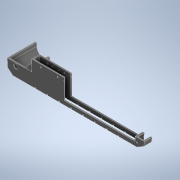
# Autodesk Inventor part: dolni-cast
Saved by Autodesk Inventor 2022 (Build 260153000, 153)
## iProperties
Created: 2022-11-08
Part Number: dolni-cast
Material: Generic
Document SubType Name: Modeling
Designer: matys
Density: 1 g/cm^3
Appearance: Gray
Author: matys
Autodesk Inventor part; units mm, degrees
ref_plane "YZ Plane" through (0, 0, 0) normal (1, 0, 0) x (0, 1, 0)
ref_plane "XZ Plane" through (0, 0, 0) normal (0, 1, 0) x (-1, 0, 0)
ref_plane "XY Plane" through (0, 0, 0) normal (0, 0, 1) x (1, 0, 0)
sketch "Sketch1" plane through (0, 0, 0) normal (0, 1, 0) x (-1, 0, 0)
  line L0 (0, 0) -> (0, -100)
  line L1 (0, 0) -> (-247.347, 0)
  line L2 (-247.347, 0) -> (-247.347, -100)
  line L3 (-247.347, -100) -> (0, -100)
  dimension "d0" = 100
  dimension "d1" = 247.347
  dimension "d2" = 100
  constraints: 8 end point, 1 horizontal, 1 perpendicular, 1 vertical
  measures "d0" distance of L0.start L0.end
  measures "d1" distance of L0.start L1.end
  measures "d2" distance of L1.end L2.end
extrude "Extrusion1" add sketch "Sketch1" along normal blind 38.0143
sketch "Sketch2" plane through (0, 0, 0) normal (0, 0, 1) x (1, 0, 0)
  line L0 (247.347, 0) -> (0, 0)
  line L1 (0, 0) -> (0, 3.5)
  line L2 (0, 0) -> (0, 38.0143)
  line L3 (247.347, 0) -> (247.347, 38.0143)
  line L4 (0, 3.5) -> (2, 3.5)
  line L5 (0, 0) -> (0, 3.5)
  line L6 (0, 3.5) -> (2, 3.5)
  line L7 (247.347, 38.0143) -> (0, 38.0143)
  arc A0 (3.965119, 16.034845) -> (16.530008, 3.5) centre (16.5, 16.034845) ccw
  line L8 (16.5, 16.034845) -> (3.965119, 16.034845)
  line L9 (2, 16.034845) -> (2, 8.034845)
  line L10 (6.849962, 8.034845) -> (14.857533, 8.034845)
  line L11 (14.857533, 8.034845) -> (6.849962, 8.034845)
  line L12 (2, 8.034845) -> (11.575556, 0)
  line L13 (2, 16.034845) -> (0, 38.0143)
  line L14 (2, 3.5) -> (7.404418, 3.5)
  line L15 (16.469992, 3.5) -> (16.530008, 3.5)
  line L16 (0, 3.5) -> (7.404418, 3.5)
  line L17 (2, 16.034845) -> (3, 16.034845)
  line L18 (1.663936, 35.652509) -> (1.493828, 38.15023)
  line L19 (3.094685, 35.782699) -> (1.663936, 35.652509)
  line L20 (0, 38.0143) -> (1.493828, 38.15023)
  line L21 (3.094685, 35.782699) -> (3.965119, 16.034845)
  line L22 (247.347, 0) -> (230.9326, 0)
  line L23 (230.9326, 0) -> (230.9326, 3.5)
  line L24 (230.9326, 3.5) -> (242.883751, 10.4)
  line L25 (231.248952, 0.023376) -> (243.200103, 6.923376)
  line L26 (243.200103, 6.923376) -> (247.347, 25.567765)
  line L27 (240.6078, 9.085979) -> (243.787005, 23.379642)
  line L28 (244.329151, 25.817122) -> (247.347, 25.817122)
  line L29 (16.469992, 3.5) -> (230.9326, 3.5)
  line L30 (237.270641, 3.5) -> (247.347, 3.5)
  line L31 (247.347, 25.567765) -> (247.347, 25.817122)
  line L32 (244.329151, 25.817122) -> (245.829151, 25.817122)
  line L33 (245.829151, 25.817122) -> (245.273551, 23.379642)
  line L34 (245.273551, 23.379642) -> (243.787005, 23.379642)
  line L35 (247.347, 25.567765) -> (247.347, 0)
  line L36 (231.208463, 0) -> (247.347, 0)
  line L37 (247.347, 25.817122) -> (247.347, 38.0143)
  line L38 (247.347, 38.0143) -> (1.503086, 38.0143)
  line L39 (0, 38.0143) -> (0, 0)
  line L40 (0, 0) -> (11.575556, 0)
  line L41 (11.575556, 0) -> (231.208463, 0)
  line L42 (231.248952, 0.023376) -> (231.208463, 0)
  point P0 (16.530008, 3.5)
  dimension "d5" = 3.5
  dimension "d9" = 2
  dimension "d12" = 8
  dimension "d13" = 12.5
  dimension "d14" = 40
  dimension "d17" = 1
  dimension "d20" = 16.4144
  dimension "d21" = 13.8
  dimension "d23" = 13.8
  dimension "d24" = 19.1
  dimension "d26" = 17.14
  dimension "d27" = 1.5
  dimension "d28" = 2.5
  constraints: 78 end point, 15 point on line, 10 collinear, 6 horizontal, 5 perpendicular, 4 point on circle, 2 parallel, 1 centre point
  measures "d5" distance of L0.end L1.end
  measures "d9" distance of L1.end L4.end
  measures "d12" distance of L9.start L9.end
  measures "d13" distance of L9.end L12.end
  measures "d14" angle of L10 L12
  measures "d17" distance of L9.start L17.end
  measures "d20" distance of L0.start L22.end
  measures "d21" distance of L23.end L24.end
  measures "d23" distance of L25.start L25.end
  measures "d24" distance of L25.end L26.end
  measures "d26" distance of L27.start L28.start
  measures "d27" distance of L28.start L32.end
  measures "d28" distance of L32.end L33.end
extrude "Extrusion2" cut sketch "Sketch2" against normal through all contours L0 L42 L25 L30 L3 | L30 L25 L26 L3 | L0 L1 L4 L14 L12 | L29 A0 L21 L19 L18 L7 L3 L28 L33 L34 L27 L24 | L14 L4 L2 L13 L9 L12
sketch "Sketch3" plane through (16.469992, 3.5, 0) normal (0, 1, 0) x (1, 0, 0)
  line L0 (226.73011, 0) -> (230.877008, 0)
  line L1 (230.877008, 0) -> (230.877008, 2)
  line L2 (230.877008, 0) -> (230.877008, 100)
  line L3 (230.877008, 2) -> (-16.469992, 2)
  line L4 (-16.469992, 100) -> (-16.469992, 0)
  line L5 (-16.469992, 0) -> (-16.469992, 2)
  line L6 (-16.469992, 0) -> (-14.966906, 0)
  line L7 (-16.469992, 0) -> (230.877008, 0)
  line L8 (230.877008, 0) -> (230.877008, 100)
  line L9 (230.877008, 100) -> (-16.469992, 100)
  line L10 (-16.469992, 100) -> (-16.469992, 98)
  line L11 (-16.469992, 98) -> (230.877008, 98)
  line L12 (230.877008, 100) -> (230.877008, 98)
  point P0 (226.73011, 0)
  dimension "d31" = 2
  dimension "d32" = 2
  constraints: 18 end point, 5 perpendicular, 5 point on line, 1 collinear
  measures "d31" distance of L0.end L1.end
  measures "d32" distance of L9.end L10.end
extrude "Extrusion3" add sketch "Sketch3" along normal blind 34.5143 contours L7 L6 L4 L3 L1 L0 | L11 L4 L9 L2
sketch "Sketch4" plane through (0, 3.5, -98) normal (0, 0, 1) x (1, 0, 0)
  line L0 (11.575556, -3.5) -> (7.404418, 0)
  line L1 (7.404418, 0) -> (2, 4.534845)
  line L2 (7.404418, 0) -> (2, 4.534845)
  line L3 (2, 4.534845) -> (2, 12.534845)
  line L4 (2, 4.534845) -> (2, 12.534845)
  line L5 (2, 12.534845) -> (0, 34.5143)
  line L6 (2, 12.534845) -> (0, 34.5143)
  line L7 (0, 0) -> (0, 34.5143)
  line L8 (0, 34.5143) -> (0, 0)
  line L9 (0, 0) -> (7.404418, 0)
  point P0 (0, -3.5)
  constraints: 10 end point, 4 collinear, 1 perpendicular
extrude "Extrusion4" cut sketch "Sketch4" along normal through all both and the other way through all
sketch "Sketch5" plane through (237.270641, 3.5, -98) normal (0, 0, 1) x (1, 0, 0)
  line L0 (0, 0) -> (5.929462, 3.423376)
  line L1 (0, 0) -> (5.929462, 3.423376)
  line L2 (5.929462, 3.423376) -> (10.076359, 22.067765)
  line L3 (5.929462, 3.423376) -> (10.076359, 22.067765)
  line L4 (0, 0) -> (10.076359, 0)
  line L5 (10.076359, 22.067765) -> (10.076359, 0)
  line L6 (10.076359, 0) -> (0, 0)
  point P0 (-237.270641, -3.5)
  constraints: 8 end point, 2 collinear, 2 perpendicular
extrude "Extrusion5" cut sketch "Sketch5" along normal through all both and the other way through all
chamfer "Chamfer1" distance 245.847 distance2 12.197 1 edges at (247.347, 38.0143, -1) measured on face at (82.95, 38.0143, -99.3333)
sketch "Sketch6" plane through (16.469992, 3.5, -98) normal (0, 0, 1) x (1, 0, 0)
  arc A0 (-12.504873, 12.534845) -> (0, 0) centre (0.030008, 12.534845) ccw
  circle A1 centre (0.030008, 12.534845) radius 12.534881
  circle A2 centre (0.030008, 12.534845) radius 12.75
  line L0 (0.030008, 12.534845) -> (12.780008, 12.534845)
  line L1 (12.780008, 12.534845) -> (12.780008, 0)
  line L2 (0, 0) -> (214.462608, 0)
  line L3 (12.780008, 0) -> (2.362422, 0)
  line L4 (12.780008, 12.534845) -> (15.780008, 12.534845)
  line L5 (15.780008, 12.534845) -> (15.780008, 0)
  line L6 (15.780008, 0) -> (14.280008, 0)
  line L7 (14.280008, 0) -> (12.780008, 0)
  point P0 (-16.469992, -3.5)
  point P1 (2.362422, 0)
  point P2 (15.780008, 0)
  dimension "d42" = 25.5
  dimension "d43" = 3
  constraints: 14 end point, 4 perpendicular, 4 point on line, 2 coincident, 2 point on circle, 1 centre point, 1 horizontal, 1 horizontal alignment, 2 other
  measures "d42" diameter of A2
  measures "d43" distance of L0.end L4.end
extrude "Extrusion6" add sketch "Sketch6" along normal through all contours A2 L1 L2 | L4 L5 L2 L1
sketch "Sketch7" plane through (29.25, 16.034845, -98) normal (0, 1, 0) x (1, 0, 0)
  line L0 (-27.746904, 0) -> (218.097, 0)
  line L1 (3, 0) -> (3, -96)
  line L2 (0.096475, 0) -> (3, 0)
  line L3 (3, -96) -> (201.6826, -96)
  line L4 (3, 0) -> (3, -96)
  line L5 (3, -96) -> (3, -48)
  line L6 (3, -48) -> (0, -48)
  line L7 (0, 0) -> (0, -96)
  line L8 (0, -48) -> (0, -43)
  line L9 (0, -43) -> (3, -43)
  line L10 (3, -48) -> (3, -53)
  line L11 (3, -53) -> (0, -53)
  line L12 (0, -53) -> (0, -48)
  line L13 (0, -43) -> (-10.417585, -43)
  line L14 (-10.417585, -96) -> (-10.417585, 0)
  line L15 (0, -53) -> (-10.417585, -53)
  line L16 (-10.417585, -53) -> (-10.417585, -43)
  point P0 (-29.25, -98)
  point P1 (-10.417585, -53)
  point P2 (3, -53)
  dimension "d46" = 48
  dimension "d47" = 5
  dimension "d48" = 5
  constraints: 24 end point, 7 point on line, 6 perpendicular, 2 midpoint
  measures "d46" distance of L1.end L5.end
  measures "d47" distance of L6.end L8.end
  measures "d48" distance of L5.end L10.end
extrude "Extrusion7" cut sketch "Sketch7" against normal blind 12.535 contours L13 L7 L15 L14 | L9 L1 L6 L7 | L6 L1 L11 L7
sketch "Sketch8" plane through (32.25, 3.5, -98) normal (0, 0, 1) x (1, 0, 0)
  arc A0 (-28.284881, 12.534845) -> (-15.780008, 0) centre (-15.75, 12.534845) ccw
  line L0 (-15.75, 12.534845) -> (-28.284881, 12.534845)
  line L1 (-28.284881, 12.534845) -> (-15.75, 12.534845)
  circle A1 centre (-15.75, 12.534845) radius 3.75
  point P0 (-32.25, -3.5)
  dimension "d51" = 7.5
  constraints: 4 end point, 1 centre point, 1 coincident, 1 collinear, 1 horizontal
  measures "d51" diameter of A1
extrude "Extrusion8" cut sketch "Sketch8" along normal through all both and the other way through all
fillet "Fillet1" radius 1 2 edges at (12.75, 16.0348, -98) (12.75, 16.0348, -2)
fillet "Fillet2" radius 2 2 edges at (26.3056, 7.8855, -55) (26.3056, 7.8855, -45)
sketch "Sketch9" plane through (11.575556, 0, 0) normal (0, 0, 1) x (1, 0, 0)
  line L0 (219.632908, 0) -> (0, 0)
  line L1 (40.927234, 0) -> (77.927234, 0)
  line L2 (77.927234, 0) -> (77.927234, 37)
  line L3 (77.927234, 37) -> (-21.111076, 37)
  circle A0 centre (4.924444, 16.034845) radius 3.75
  circle A1 centre (4.924444, 16.034845) radius 4.75
  line L4 (4.924444, 16.034845) -> (4.924444, 12.284845)
  arc A2 (-7.610437, 16.034845) -> (4.894437, 3.5) centre (4.924444, 16.034845) ccw
  line L5 (4.924444, 16.034845) -> (4.924444, 1.034845)
  line L6 (4.924444, 1.034845) -> (39.924444, 1.034845)
  circle A3 centre (39.924444, 1.034845) radius 1.1
  line L7 (39.924444, 1.034845) -> (39.924444, 37)
  line L8 (39.924444, 37) -> (51.574444, 37)
  line L9 (51.574444, 37) -> (39.924444, 37)
  line L10 (-10.072459, 38.014146) -> (235.771444, 25.8173)
  line L11 (39.924444, 37) -> (21.524444, 37)
  line L12 (21.524444, 37) -> (15.524444, 37)
  line L13 (15.524444, 37) -> (15.524444, 32)
  line L14 (15.524444, 32) -> (51.574444, 32)
  line L15 (51.574444, 32) -> (57.574444, 32)
  line L16 (57.574444, 32) -> (57.574444, 42)
  line L17 (57.574444, 42) -> (15.524444, 42)
  line L18 (15.524444, 42) -> (15.524444, 37)
  line L19 (219.357044, 3.5) -> (20.674444, 3.5)
  line L20 (39.924444, 1.034845) -> (60.924444, 1.034845)
  circle A4 centre (60.924444, 1.034845) radius 1.1
  circle A5 centre (81.924444, 1.034845) radius 1.1
  circle A6 centre (102.924444, 1.034845) radius 1.1
  circle A7 centre (123.924444, 1.034845) radius 1.1
  circle A8 centre (144.924444, 1.034845) radius 1.1
  circle A9 centre (165.912921, 1.034845) radius 1.1
  circle A10 centre (186.903317, 1.034845) radius 1.1
  line L21 (39.924444, 37) -> (51.574444, 37)
  line L22 (39.924444, 37) -> (28.274444, 37)
  line L23 (28.274444, 37) -> (39.924444, 1.034845)
  circle A11 centre (28.274444, 37) radius 1.1
  line L24 (21.524444, 37) -> (39.924444, 37)
  line L25 (58.324444, 37) -> (39.924444, 1.034845)
  circle A12 centre (58.324444, 37) radius 1.1
  line L26 (49.274444, 37) -> (60.924444, 1.034845)
  circle A13 centre (49.274444, 37) radius 1.1
  line L27 (79.324444, 37) -> (60.924444, 1.034845)
  circle A14 centre (79.324444, 37) radius 1.1
  line L28 (70.274444, 37) -> (81.924444, 1.034845)
  circle A15 centre (70.274444, 37) radius 1.1
  line L29 (100.324444, 37) -> (81.924444, 1.034845)
  circle A16 centre (100.324444, 37) radius 1.1
  line L30 (91.274444, 37) -> (102.924444, 1.034845)
  circle A17 centre (91.274444, 37) radius 1.1
  line L31 (121.324444, 37) -> (102.924444, 1.034845)
  circle A18 centre (121.324444, 37) radius 1.1
  line L32 (112.274444, 37) -> (123.924444, 1.034845)
  circle A19 centre (112.274444, 37) radius 1.1
  line L33 (142.324444, 37) -> (123.924444, 1.034845)
  circle A20 centre (142.324444, 37) radius 1.1
  line L34 (133.274444, 37) -> (144.924444, 1.034845)
  circle A21 centre (133.274444, 37) radius 1.1
  line L35 (163.324444, 37) -> (144.924444, 1.034845)
  circle A22 centre (163.324444, 37) radius 1.1
  line L36 (154.262921, 37) -> (165.912921, 1.034845)
  circle A23 centre (154.262921, 37) radius 1.1
  line L37 (184.312921, 37) -> (165.912921, 1.034845)
  circle A24 centre (184.312921, 37) radius 1.1
  line L38 (175.253317, 37) -> (186.903317, 1.034845)
  circle A25 centre (175.253317, 37) radius 1.1
  line L39 (205.303317, 37) -> (186.903317, 1.034845)
  circle A26 centre (205.303317, 37) radius 1.1
  line L40 (15.524444, 42) -> (14.524444, 42)
  line L41 (14.524444, 42) -> (14.524444, 32)
  line L42 (14.524444, 32) -> (15.524444, 32)
  point P0 (-11.575556, 0)
  dimension "d56" = 37
  dimension "d59" = 15
  dimension "d60" = 35
  dimension "d61" = 2.2
  dimension "d62" = 11.65
  dimension "d66" = 18.4
  dimension "d68" = 6
  dimension "d69" = 5
  dimension "d70" = 6
  dimension "d71" = 10
  dimension "d73" = 21
  dimension "d74" = 2.2
  dimension "d113" = 2.2
  dimension "d116" = 2.2
  dimension "d119" = 2.2
  dimension "d122" = 2.2
  dimension "d125" = 2.2
  dimension "d128" = 2.2
  dimension "d184" = 2.2
  dimension "d185" = 2.2
  dimension "d186" = 2.2
  dimension "d187" = 2.2
  dimension "d188" = 2.2
  dimension "d189" = 2.2
  dimension "d190" = 2.2
  dimension "d191" = 2.2
  dimension "d192" = 1
  dimension "d193" = 10
  constraints: 80 end point, 27 coincident, 24 centre point, 9 perpendicular, 9 point on line, 3 collinear, 3 horizontal, 2 symmetric about line, 1 vertical, 1 vertical alignment, 1 other
  measures "d56" distance of L1.start L1.end
  measures "d59" distance of L5.start L5.end
  measures "d60" distance of L5.end L6.end
  measures "d61" diameter of A3
  measures "d62" distance of L7.end L8.end
  measures "d66" distance of L7.end L11.end
  measures "d68" distance of L12.start L12.end
  measures "d69" distance of L12.end L13.end
  measures "d70" distance of L14.end L15.end
  measures "d71" distance of L15.end L16.end
  measures "d73" distance of L7.start L20.end
  measures "d74" diameter of A4
  measures "d113" diameter of A5
  measures "d116" diameter of A6
  measures "d119" diameter of A7
  measures "d122" diameter of A8
  measures "d125" diameter of A9
  measures "d128" diameter of A10
  measures "d184" diameter of A12
  measures "d185" diameter of A14
  measures "d186" diameter of A16
  measures "d187" diameter of A18
  measures "d188" diameter of A20
  measures "d189" diameter of A22
  measures "d190" diameter of A24
  measures "d191" diameter of A26
  measures "d192" distance of L17.end L40.end
  measures "d193" distance of L40.end L41.end
sketch "Sketch10" plane through (230.9326, 3.5, -2) normal (0, 1, 0) x (1, 0, 0)
  line L0 (-198.6826, 0) -> (-198.6826, -2)
  line L1 (-198.6826, -2) -> (-198.6826, 0)
  line L2 (-198.6826, 43) -> (-198.6826, 0)
  line L3 (-198.6826, 0) -> (-198.6826, 10)
  line L4 (-198.6826, 10) -> (-198.6826, 12)
  line L5 (-198.6826, 12) -> (-198.6826, 22)
  line L6 (-198.6826, 22) -> (-198.6826, 24)
  line L7 (-198.6826, 24) -> (9.292575, 24)
  line L8 (0, 0) -> (0, 96)
  line L9 (0, 24) -> (0, 0)
  line L10 (0, 0) -> (-198.6826, 0)
  point P0 (-230.9326, -2)
  dimension "d77" = 10
  dimension "d78" = 2
  dimension "d79" = 10
  dimension "d80" = 2
  constraints: 18 end point, 6 point on line, 2 collinear, 2 perpendicular, 1 vertical
  measures "d77" distance of L0.start L3.end
  measures "d78" distance of L3.end L4.end
  measures "d79" distance of L4.end L5.end
  measures "d80" distance of L5.end L6.end
extrude "Extrusion9" add sketch "Sketch10" along normal blind 38.5
sketch "Sketch11" plane through (32.25, 42, -2) normal (0, 0, 1) x (1, 0, 0)
  line L0 (0, 0) -> (-5.15, 0)
  line L1 (-5.15, 0) -> (-5.15, -5.255771)
  line L2 (-30.746904, -3.985854) -> (215.097, -16.1827)
  line L3 (-5.15, -5.255771) -> (0, -5.511274)
  line L4 (0, -5.511274) -> (199.767396, -15.422165)
  line L5 (0, 0) -> (198.6826, 0)
  line L6 (198.6826, -15.368346) -> (198.6826, 0)
  line L7 (198.6826, 0) -> (198.6826, -15.368346)
  line L8 (198.6826, -15.368346) -> (198.6826, 0)
  line L9 (198.6826, 0) -> (-5.15, 0)
  line L10 (-5.15, 0) -> (-6.15, 0)
  line L11 (0, -5.511274) -> (0, 0)
  line L12 (-6.15, 0) -> (-6.15, -5.206159)
  line L13 (-5.15, -5.255771) -> (-6.15, -5.206159)
  line L14 (0, -5.511274) -> (-30.746904, -3.985854)
  point P0 (-32.25, -42)
  dimension "d83" = 5.15
  dimension "d104" = 1
  constraints: 20 end point, 4 point on line, 3 collinear, 3 perpendicular, 1 horizontal, 1 vertical
  measures "d83" distance of L0.start L0.end
  measures "d104" distance of L0.end L10.end
extrude "Extrusion10" add sketch "Sketch11" along normal blind 2
sketch "Sketch13" plane through (230.9326, 3.5, -26) normal (0, 0, -1) x (-1, 0, 0)
  line L0 (204.8326, 28.5) -> (204.8326, 38.5) projected
  line L1 (204.8326, 38.5) -> (204.8326, 33.5)
  line L2 (204.8326, 33.5) -> (0, 33.5)
  line L3 (0, 0) -> (0, 38.5) projected
  line L4 (204.8326, 33.5) -> (191.0826, 33.5)
  circle A0 centre (191.0826, 33.5) radius 1.1
  line L5 (191.0826, 33.5) -> (161.0326, 33.5)
  circle A1 centre (161.0326, 33.5) radius 1.1
  line L6 (161.0326, 33.5) -> (170.0826, 33.5)
  circle A2 centre (170.0826, 33.5) radius 1.1
  line L7 (170.0826, 33.5) -> (140.0326, 33.5)
  line L8 (140.0326, 33.5) -> (149.0826, 33.5)
  circle A3 centre (149.0826, 33.5) radius 1.1
  circle A4 centre (149.0826, 33.5) radius 1.1
  circle A5 centre (140.0326, 33.5) radius 1.1
  circle A6 centre (149.0826, 33.5) radius 1.1
  circle A7 centre (119.0326, 33.5) radius 1.1
  circle A8 centre (128.0826, 33.5) radius 1.1
  circle A9 centre (98.0326, 33.5) radius 1.1
  circle A10 centre (107.0826, 33.5) radius 1.1
  circle A11 centre (77.0326, 33.5) radius 1.1
  circle A12 centre (86.0826, 33.5) radius 1.1
  circle A13 centre (56.0326, 33.5) radius 1.1
  circle A14 centre (65.0826, 33.5) radius 1.1
  circle A15 centre (35.0326, 33.5) radius 1.1
  circle A16 centre (44.0826, 33.5) radius 1.1
  circle A17 centre (14.0326, 33.5) radius 1.1
  point P0 (230.9326, -3.5)
  point P1 (147.9826, 33.5)
  point P2 (150.1826, 33.5)
  dimension "d194" = 13.75
  dimension "d195" = 2.2
  dimension "d196" = 30.05
  dimension "d197" = 9.05
  dimension "d198" = 2.2
  dimension "d199" = 30.05
  dimension "d200" = 9.05
  dimension "d201" = 2.2
  dimension "d202" = 2.2
  dimension "d203" = 2.2
  dimension "d204" = 2.2
  dimension "d205" = 2.2
  dimension "d206" = 2.2
  dimension "d207" = 2.2
  dimension "d208" = 2.2
  dimension "d209" = 2.2
  dimension "d210" = 2.2
  dimension "d211" = 2.2
  dimension "d212" = 2.2
  dimension "d213" = 2.2
  dimension "d214" = 2.2
  constraints: 18 centre point, 14 end point, 6 point on line, 5 coincident, 1 midpoint, 1 perpendicular
  measures "d194" distance of L1.end L4.end
  measures "d195" diameter of A0
  measures "d196" distance of L5.start L5.end
  measures "d197" distance of L6.start L6.end
  measures "d198" diameter of A2
  measures "d199" distance of L7.start L7.end
  measures "d200" distance of L7.end L8.end
  measures "d201" diameter of A4
  measures "d202" diameter of A5
  measures "d203" diameter of A6
  measures "d204" diameter of A7
  measures "d205" diameter of A8
  measures "d206" diameter of A9
  measures "d207" diameter of A10
  measures "d208" diameter of A11
  measures "d209" diameter of A12
  measures "d210" diameter of A13
  measures "d211" diameter of A14
  measures "d212" diameter of A15
  measures "d213" diameter of A16
  measures "d214" diameter of A17
extrude "Extrusion12" cut sketch "Sketch13" against normal blind 14 contours A0 L2 | L2 A0 | A1 L2 | L2 A1 | A3 L2 | L2 A3 | A7 L2 | L2 A7 | A10 L2 | L2 A10 | A11 L2 | L2 A11 | A14 L2 | L2 A14 | A15 L2 | L2 A15
sketch "Sketch14" plane through (230.9326, 42, -2) normal (0, 1, 0) x (1, 0, 0)
  line L0 (-196.7326, 24) -> (-196.7326, -2) projected
  line L1 (0, 24) -> (-198.6826, 24) projected
  line L2 (-204.8326, 24) -> (-204.8326, 22)
  line L3 (-204.8326, 0) -> (-204.8326, 24) projected
  line L4 (-204.8326, 22) -> (-197.8326, 22)
  line L5 (-204.8326, 22) -> (-203.8326, 22)
  line L6 (-203.8326, 22) -> (-203.8326, 12)
  line L7 (-201.6826, 96) -> (-201.6826, 55) projected
  line L8 (-203.8326, 12) -> (-193.8326, 12)
  line L9 (-193.8326, 12) -> (-193.8326, 22)
  line L10 (-193.8326, 22) -> (-197.8326, 22)
  line L11 (-201.6826, 24) -> (-204.8326, 24) projected
  line L12 (-204.8326, 24) -> (-167.7826, 24)
  line L13 (-167.7826, 24) -> (-167.7826, 11)
  line L14 (-193.8326, 22) -> (-167.7826, 22)
  line L15 (-167.7826, 22) -> (-161.7826, 22)
  line L16 (-161.7826, 22) -> (-161.7826, 12)
  line L17 (-161.7826, 12) -> (-193.8326, 12)
  line L18 (-161.7826, 22) -> (0, 22)
  line L19 (-197.8326, 22) -> (-167.7826, 22)
  line L20 (-167.7826, 22) -> (-155.8326, 22)
  line L21 (-197.8326, 22) -> (-155.8326, 22)
  line L22 (-155.8326, 22) -> (-125.7826, 22)
  line L23 (-125.7826, 22) -> (-125.7826, 12)
  line L24 (-125.7826, 12) -> (-161.7826, 12)
  line L25 (-125.7826, 22) -> (-113.8326, 22)
  line L26 (-113.8326, 22) -> (-113.8326, 12)
  line L27 (-113.8326, 12) -> (-125.7826, 12)
  line L28 (-113.8326, 22) -> (-83.7826, 22)
  line L29 (-83.7826, 22) -> (-83.7826, 12)
  line L30 (-83.7826, 12) -> (-113.8326, 12)
  line L31 (-83.7826, 22) -> (-71.8326, 22)
  line L32 (-71.8326, 22) -> (-71.8326, 12)
  line L33 (-71.8326, 12) -> (-83.7826, 12)
  line L34 (-71.8326, 22) -> (-41.7826, 22)
  line L35 (-41.7826, 22) -> (-41.7826, 12)
  line L36 (-41.7826, 12) -> (-71.8326, 12)
  line L37 (-41.7826, 22) -> (-34.7826, 22)
  line L38 (-34.7826, 22) -> (-34.7826, 12)
  line L39 (-34.7826, 12) -> (-41.7826, 12)
  line L40 (-34.7826, 12) -> (-27.7826, 12)
  line L41 (-27.7826, 12) -> (-27.7826, 22)
  point P0 (-230.9326, -2)
  point P1 (-201.6826, 0)
  dimension "d105" = 7
  dimension "d106" = 1
  dimension "d109" = 10
  dimension "d110" = 37.05
  dimension "d111" = 6
  dimension "d112" = 10
  dimension "d131" = 11.95
  dimension "d132" = 30.05
  dimension "d133" = 11.95
  dimension "d134" = 30.05
  dimension "d135" = 11.95
  dimension "d136" = 30.05
  dimension "d137" = 7
  dimension "d215" = 7
  constraints: 72 end point, 18 perpendicular, 10 point on line, 3 collinear, 2 horizontal, 1 vertical, 11 other
  measures "d105" distance of L2.end L4.end
  measures "d106" distance of L2.end L5.end
  measures "d109" distance of L6.end L8.end
  measures "d110" distance of L2.start L12.end
  measures "d111" distance of L14.end L15.end
  measures "d112" distance of L15.end L16.end
  measures "d131" distance of L14.end L20.end
  measures "d132" distance of L20.end L22.end
  measures "d133" distance of L22.end L25.end
  measures "d134" distance of L25.end L28.end
  measures "d135" distance of L28.end L31.end
  measures "d136" distance of L31.end L34.end
  measures "d137" distance of L34.end L37.end
  measures "d215" distance of L38.end L40.end
extrude "Extrusion13" cut sketch "Sketch14" against normal through all contours L10 L9 L8 L0 | L0 L8 L6 L4 L10 | L14 L13 L17 L9 | L15 L16 L17 L13 | L18 L23 L24 L16 | L23 L18 L26 L27 | L26 L18 L29 L30 | L29 L18 L32 L33 | L32 L18 L35 L36 | L35 L18 L38 L39 | L38 L18 L41 L40
sketch "Sketch15" plane through (230.9326, 42, -2) normal (0, 1, 0) x (1, 0, 0)
  line L0 (-219.357044, -2) -> (0.275863, -2)
  line L1 (-204.8326, -2) -> (-204.8326, 12)
  line L2 (-204.8326, 12) -> (-204.8326, -2)
  line L3 (-204.8326, 0) -> (-201.6826, 0)
  line L4 (-204.8326, -2) -> (-204.8326, 0)
  line L5 (-204.8326, 0) -> (-204.8326, 12)
  line L6 (-34.7826, 12) -> (-203.8326, 12)
  line L7 (-204.8326, 12) -> (-203.8326, 12)
  line L8 (-203.8326, 12) -> (-203.8326, 10)
  line L9 (-203.8326, 10) -> (0.275863, 10)
  line L10 (0.275863, 98) -> (0.275863, -2)
  line L11 (-203.8326, 10) -> (-203.8326, 0)
  line L12 (-203.8326, 0) -> (0.275863, 0)
  line L13 (0.275863, 0) -> (0.275863, 10)
  line L14 (-203.8326, 0) -> (-197.8326, 0)
  line L15 (-197.8326, 0) -> (-176.8326, 0)
  line L16 (-176.8326, 0) -> (-146.7826, 0)
  line L17 (-146.7826, 0) -> (-146.7826, 10)
  line L18 (-176.8326, 0) -> (-176.8326, 10)
  line L19 (-146.7826, 0) -> (-134.8326, 0)
  line L20 (-134.8326, 0) -> (-104.7826, 0)
  line L21 (-104.7826, 0) -> (-104.7826, 10)
  line L22 (-104.7826, 0) -> (-92.8326, 0)
  line L23 (-92.8326, 0) -> (-62.7826, 0)
  line L24 (-62.7826, 0) -> (-50.8326, 0)
  line L25 (-50.8326, 0) -> (-20.7826, 0)
  line L26 (-20.7826, 0) -> (-20.7826, 10)
  line L27 (-20.7826, 0) -> (-13.7826, 0)
  line L28 (-13.7826, 0) -> (-13.7826, 10)
  line L29 (-176.8326, 0) -> (-183.8326, 0)
  line L30 (-183.8326, 0) -> (-183.8326, 10)
  line L31 (-13.7826, 10) -> (-6.7826, 10)
  line L32 (-6.7826, 10) -> (-6.7826, 0)
  line L33 (-13.7826, 0) -> (-6.7826, 0)
  point P0 (-230.9326, -2)
  dimension "d142" = 2
  dimension "d143" = 10
  dimension "d144" = 6
  dimension "d145" = 21
  dimension "d146" = 30.05
  dimension "d147" = 11.95
  dimension "d148" = 30.05
  dimension "d149" = 11.95
  dimension "d150" = 30.05
  dimension "d151" = 11.95
  dimension "d152" = 30.05
  dimension "d153" = 7
  dimension "d156" = 7
  dimension "d235" = 7
  constraints: 56 end point, 11 vertical, 4 point on line, 2 collinear, 2 horizontal, 2 perpendicular, 24 other
  measures "d142" distance of L6.end L8.end
  measures "d143" distance of L8.end L11.end
  measures "d144" distance of L11.end L14.end
  measures "d145" distance of L14.end L15.end
  measures "d146" distance of L15.end L16.end
  measures "d147" distance of L16.end L19.end
  measures "d148" distance of L19.end L20.end
  measures "d149" distance of L20.end L22.end
  measures "d150" distance of L22.end L23.end
  measures "d151" distance of L23.end L24.end
  measures "d152" distance of L24.end L25.end
  measures "d153" distance of L25.end L27.end
  measures "d156" distance of L15.end L29.end
  measures "d235" distance of L28.end L31.end
extrude "Extrusion14" cut sketch "Sketch15" against normal through all contours L12 L28 L9 L32 | L12 L26 L9 L28 | L9 L18 L12 L30 | L12 L21 L9 L26 | L9 L17 L12 L18 | L9 L21 L12 L17
sketch "Sketch16" plane through (11.575556, 0, 0) normal (0, 0, 1) x (1, 0, 0)
  line L0 (219.357044, 42) -> (14.524444, 42)
  line L1 (14.524444, 42) -> (21.524444, 42)
  line L2 (21.524444, 42) -> (51.574444, 42)
  line L3 (20.674444, 42) -> (191.574444, 42)
  line L4 (21.524444, 42) -> (39.924444, 42)
  line L5 (39.924444, 42) -> (39.924444, 1)
  circle A0 centre (39.924444, 1) radius 1.1
  line L6 (39.924444, 1) -> (60.924444, 1)
  line L7 (60.924444, 1) -> (81.924444, 1)
  line L8 (81.924444, 1) -> (102.924444, 1)
  line L9 (102.924444, 1) -> (123.924444, 1)
  line L10 (123.924444, 1) -> (144.924444, 1)
  line L11 (144.924444, 1) -> (165.924444, 1)
  line L12 (165.924444, 1) -> (186.924444, 1)
  line L13 (39.924444, 1) -> (186.924444, 1) construction
  line L14 (35.524444, 0) -> (212.574444, 0)
  line L15 (39.924444, -6.5) -> (186.924444, -6.5)
  line L16 (186.924444, 8.5) -> (39.924444, 8.5)
  arc A1 (39.924444, 8.5) -> (39.924444, -6.5) centre (39.924444, 1) ccw
  arc A2 (186.924444, -6.5) -> (186.924444, 8.5) centre (186.924444, 1) ccw
  line L17 (194.424444, 1) -> (194.424444, -6.5)
  line L18 (194.424444, -6.5) -> (186.924444, -6.5)
  line L19 (194.424444, 1) -> (194.424444, 8.5)
  line L20 (194.424444, 8.5) -> (186.924444, 8.5)
  circle A3 centre (60.924444, 1) radius 1.1
  circle A4 centre (81.924444, 1) radius 1.1
  circle A5 centre (102.924444, 1) radius 1.1
  circle A6 centre (123.924444, 1) radius 1.1
  circle A7 centre (144.924444, 1) radius 1.1
  circle A8 centre (165.924444, 1) radius 1.1
  circle A9 centre (186.924444, 1) radius 1.1
  point P0 (-11.575556, 0)
  point P1 (15.524444, 42)
  point P2 (184.574444, 42)
  point P3 (205.574444, 0)
  point P4 (113.424444, 1)
  point P5 (194.424444, 0)
  point P6 (194.357479, 0)
  dimension "d167" = 7
  dimension "d168" = 30.05
  dimension "d169" = 18.4
  dimension "d170" = 41
  dimension "d171" = 2.2
  dimension "d172" = 21
  dimension "d173" = 21
  dimension "d174" = 21
  dimension "d175" = 21
  dimension "d176" = 21
  dimension "d177" = 21
  dimension "d178" = 21
  dimension "d179" = 15
  dimension "d255" = 2.2
  dimension "d256" = 2.2
  dimension "d257" = 2.2
  dimension "d258" = 2.2
  dimension "d259" = 2.2
  dimension "d260" = 2.2
  dimension "d261" = 2.2
  constraints: 38 end point, 10 centre point, 10 point on line, 6 tangent, 5 point on circle, 2 parallel, 1 coincident, 1 collinear, 1 horizontal, 1 midpoint, 1 perpendicular, 1 vertical
  measures "d167" distance of L0.end L1.end
  measures "d168" distance of L1.end L2.end
  measures "d169" distance of L1.end L4.end
  measures "d170" distance of L4.end L5.end
  measures "d171" diameter of A0
  measures "d172" distance of L6.start L6.end
  measures "d173" distance of L6.end L7.end
  measures "d174" distance of L7.end L8.end
  measures "d175" distance of L8.end L9.end
  measures "d176" distance of L9.end L10.end
  measures "d177" distance of L10.end L11.end
  measures "d178" distance of L11.end L12.end
  measures "d179" diameter of A2
  measures "d255" diameter of A3
  measures "d256" diameter of A4
  measures "d257" diameter of A5
  measures "d258" diameter of A6
  measures "d259" diameter of A7
  measures "d260" diameter of A8
  measures "d261" diameter of A9
extrude "Extrusion15" cut sketch "Sketch16" against normal blind 14 contours A0 L6 L5 | L5 L6 A0 L14 | L14 A0 | A3 L7 L6 | L6 L7 A3 L14 | L14 A3 | A9 L14 | L14 A9 | A4 L8 L7 | L7 L8 A4 L14 | L14 A4 | A8 L14 | L14 A8 L11 L12 | A5 L9 L8 | L8 L9 A5 L14 | L12 L11 A8 | L14 A5 | A7 L14 | L14 A7 L10 L11 | A6 L10 L9 | L9 L10 A6 L14 | L11 L10 A7 | L14 A6
sketch "Sketch17" plane through (203.15, 42, -14) normal (0, 0, -1) x (-1, 0, 0)
  line L0 (170.9, 0) -> (177.05, 0)
  line L1 (170.9, 0) -> (170.9, -42)
  line L2 (176.05, -42) -> (47.108258, -42)
  line L3 (0, 0) -> (170.9, 0)
  line L4 (170.9, 0) -> (170.9, -5)
  line L5 (170.9, 0) -> (170.9, -25.965155)
  line L6 (170.9, -5) -> (169.3, -5)
  line L7 (169.3, -5) -> (169.3, 0)
  line L8 (169.3, 0) -> (170.9, 0)
  line L9 (169.3, -5) -> (169.3, -42)
  line L10 (169.3, -42) -> (170.9, -42)
  point P0 (203.15, -42)
  point P1 (159.083034, -42)
  dimension "d216" = 5
  dimension "d217" = 1.6
  constraints: 14 end point, 4 perpendicular, 3 point on line, 1 vertical
  measures "d216" distance of L0.start L4.end
  measures "d217" distance of L4.end L6.end
extrude "Extrusion16" add sketch "Sketch17" along normal blind 10
sketch "Sketch18" plane through (32.25, 0, -14) normal (0, 0, -1) x (-1, 0, 0)
  line L0 (0, 16.034845) -> (0, 0)
  line L1 (0, 0) -> (0, 16.034845)
  line L2 (0, 16.034845) -> (3, 16.034845)
  line L3 (0, 16.034845) -> (3, 16.034845)
  line L4 (3, 16.034845) -> (0, 16.034845)
  line L5 (0, 0) -> (5.15, 0)
  line L6 (5.15, 8.949473) -> (5.15, 0)
  line L7 (5.15, 0) -> (5.15, 8.949473)
  arc A0 (3, 16.034845) -> (5.15, 8.949473) centre (15.75, 16.034845) ccw
  arc A1 (3, 16.034845) -> (5.15, 8.949473) centre (15.75, 16.034845) ccw
  point P0 (32.25, 0)
  constraints: 10 end point, 2 collinear, 2 point on circle, 1 centre point, 1 perpendicular, 1 vertical
extrude "Extrusion17" add sketch "Sketch18" along normal blind 10
sketch "Sketch19" plane through (2, 8.034845, 0) normal (0, 0, 1) x (1, 0, 0)
  line L0 (24.1, 33.965155) -> (24.1, 28.758996)
  line L1 (24.1, 33.965155) -> (24.1, 28.965155)
  line L2 (24.1, 28.965155) -> (31.1, 28.965155)
  line L3 (31.1, 28.965155) -> (49.5, 28.965155)
  circle A0 centre (37.85, 28.965155) radius 1.1
  line L4 (49.5, 28.965155) -> (37.85, 28.965155)
  line L5 (37.85, 28.965155) -> (49.5, 28.965155)
  line L6 (49.5, 28.965155) -> (67.9, 28.965155)
  line L7 (67.9, 28.965155) -> (58.85, 28.965155)
  line L8 (58.85, 28.965155) -> (88.9, 28.965155)
  circle A1 centre (88.9, 28.965155) radius 1.1
  circle A2 centre (58.85, 28.965155) radius 1.1
  line L9 (88.9, 28.965155) -> (100.85, 28.965155)
  circle A3 centre (100.85, 28.965155) radius 1.1
  circle A4 centre (130.9, 28.965155) radius 1.1
  circle A5 centre (100.85, 28.965155) radius 1.1
  circle A6 centre (142.85, 28.965155) radius 1.1
  circle A7 centre (172.9, 28.965155) radius 1.1
  circle A8 centre (142.85, 28.965155) radius 1.1
  circle A9 centre (184.85, 28.965155) radius 1.1
  circle A10 centre (214.9, 28.965155) radius 1.1
  circle A11 centre (184.85, 28.965155) radius 1.1
  circle A12 centre (226.85, 28.965155) radius 1.1
  point P0 (-2, -8.034845)
  dimension "d222" = 5
  dimension "d223" = 7
  dimension "d224" = 18.4
  dimension "d225" = 18.4
  dimension "d226" = 9.05
  dimension "d227" = 30.05
  dimension "d228" = 2.2
  dimension "d229" = 11.95
  dimension "d230" = 2.2
  dimension "d231" = 2.2
  dimension "d232" = 2.2
  constraints: 18 end point, 12 centre point, 4 point on line, 3 coincident, 2 horizontal, 1 perpendicular
  measures "d222" distance of L0.start L1.end
  measures "d223" distance of L1.end L2.end
  measures "d224" distance of L2.end L3.end
  measures "d225" distance of L3.end L6.end
  measures "d226" distance of L6.end L7.end
  measures "d227" distance of L7.end L8.end
  measures "d228" diameter of A1
  measures "d229" distance of L9.start L9.end
  measures "d230" diameter of A4
  measures "d231" diameter of A7
  measures "d232" diameter of A10
extrude "Extrusion18" cut sketch "Sketch19" against normal blind 14 contours L6 A2 | L6 A2 | A1 L9 L8 | L8 L9 A1 | A3 | A4 | A6 | A7 | A9 | A10
sketch "Sketch20" plane through (230.9326, 42, -2) normal (0, 1, 0) x (1, 0, 0)
  line L0 (-27.7826, 12) -> (-197.0826, 12)
  line L1 (-27.7826, 12) -> (0, 12)
  line L2 (0, 0) -> (0, 24)
  line L3 (-27.7826, 22) -> (-27.7826, 12)
  line L4 (-27.7826, 12) -> (-24.7826, 12)
  line L5 (-24.999566, 12) -> (-27.7826, 12)
  line L6 (-24.7826, 12) -> (-24.7826, 24)
  line L7 (-198.6826, 24) -> (0, 24)
  line L8 (-24.7826, 24) -> (0, 24)
  line L9 (0, 24) -> (0, 12)
  point P0 (-230.9326, -2)
  point P1 (-24.7826, 12)
  dimension "d236" = 3
  constraints: 10 end point, 2 perpendicular, 2 point on line, 1 horizontal, 1 midpoint
  measures "d236" distance of L0.start L4.end
extrude "Extrusion19" cut sketch "Sketch20" against normal blind 38.5
sketch "Sketch22" plane through (18.832415, 3.5, -2) normal (0, 0, -1) x (-1, 0, 0)
  line L0 (17.329318, 34.514146) -> (17.168479, 32.152509)
  line L1 (17.329318, 34.514146) -> (-228.514585, 22.3173)
  line L2 (17.329318, 34.514146) -> (-228.514585, 22.3173)
  line L3 (-212.100185, 38.5) -> (-7.267585, 38.5)
  line L4 (-7.267585, 38.5) -> (-7.267585, 33.293841)
  line L5 (-7.267585, 38.5) -> (-7.267585, 33.293841)
  line L6 (-7.267585, 33.293841) -> (17.329318, 34.514146)
  line L7 (-7.267585, 33.293841) -> (-13.417585, 32.988726)
  line L8 (-13.417585, 38.5) -> (-13.417585, 12.534845)
  line L9 (-13.417585, 38.5) -> (-13.417585, 32.988726)
  line L10 (-13.417585, 38.5) -> (-7.267585, 38.5)
  line L11 (-13.417585, 38.5) -> (-7.267585, 38.5)
  point P0 (18.832415, -3.5)
  point P1 (-13.417585, 32.988726)
  constraints: 10 end point, 2 collinear, 2 point on line, 1 horizontal, 1 vertical
extrude "Extrusion20" cut sketch "Sketch22" against normal blind 38.5
sketch "Sketch23" plane through (2, 8.034845, 0) normal (0, 0, 1) x (1, 0, 0)
  circle A0 centre (14.5, 8) radius 3.75
  line L0 (14.5, 8) -> (14.5, -7)
  line L1 (14.5, -7) -> (229.208463, -7)
  line L2 (229.208463, -7) -> (229.208463, -1)
  circle A1 centre (229.208463, -1) radius 1.1
  point P0 (-2, -8.034845)
  dimension "d241" = 15
  dimension "d242" = 6
  dimension "d243" = 2.2
  constraints: 6 end point, 1 centre point, 1 coincident, 1 horizontal, 1 perpendicular, 1 vertical
  measures "d241" distance of L0.start L0.end
  measures "d242" distance of L1.end L2.end
  measures "d243" diameter of A1
extrude "Extrusion21" cut sketch "Sketch23" against normal through all contours A1
sketch "Sketch24" plane through (230.9326, 42, -14) normal (0, 0, -1) x (-1, 0, 0)
  circle A0 centre (-0.275863, -34.965155) radius 1.1
  line L0 (-0.275863, -34.965155) -> (1.224137, -34.965155)
  arc A1 (0, -36.030002) -> (0, -33.900308) centre (-0.275863, -34.965155) ccw
  line L1 (1.224137, -34.965155) -> (-0.275863, -34.965155)
  line L2 (-0.275863, -34.965155) -> (0, -38.5)
  line L3 (0, -38.5) -> (3.849587, -38.5)
  line L4 (0, -38.5) -> (24.7826, -38.5)
  line L5 (1.224137, -34.965155) -> (1.224137, -38.5)
  line L6 (1.224137, -34.965155) -> (1.224137, -32.965155)
  line L7 (1.224137, -32.965155) -> (0, -32.965155)
  line L8 (0, -38.5) -> (0, -36.030002)
  line L9 (0, -32.965155) -> (0, -38.5)
  point P0 (230.9326, -42)
  dimension "d246" = 1.5
  dimension "d247" = 2
  constraints: 16 end point, 3 perpendicular, 3 point on line, 2 horizontal
  measures "d246" distance of L0.start L0.end
  measures "d247" distance of L0.end L6.end
extrude "Extrusion22" cut sketch "Sketch24" against normal blind 12 contours L0 L5 L3 L8 A0 | A0 L9 L7 L6 L0
chamfer "Chamfer2" distance 5 distance2 1.224 1 edges at (230.9326, 9.0348, -8)
sketch "Sketch25" plane through (230.9326, 42, -2) normal (0, 1, 0) x (1, 0, 0)
  line L0 (-230.9326, 98) -> (-230.9326, -2)
  line L1 (-230.9326, -2) -> (-230.9326, 98)
  line L2 (-230.9326, 98) -> (-230.9326, 48)
  line L3 (-230.9326, 48) -> (0, 48)
  line L4 (0, 0) -> (0, 96)
  line L5 (-198.6826, 53) -> (-198.6826, 43)
  line L6 (-198.6826, 43) -> (-198.6826, 24)
  line L7 (-198.6826, 48) -> (-198.6826, 24)
  line L8 (-24.7826, 12) -> (-24.7826, 24)
  line L9 (-198.6826, 24) -> (-24.7826, 24)
  line L10 (-24.7826, 24) -> (-24.7826, 12)
  line L11 (-24.7826, 12) -> (16.4144, 11.563732)
  line L12 (16.4144, 96) -> (16.4144, 0)
  line L13 (16.4144, 11.563732) -> (16.4144, 98)
  line L14 (16.4144, 98) -> (-230.9326, 98)
  line L15 (-24.7826, 12) -> (-198.6826, 12)
  line L16 (-198.6826, 12) -> (-198.6826, 24)
  line L17 (-183.8326, 10) -> (-183.8326, 0)
  line L18 (-183.8326, 0) -> (-183.8326, 24)
  line L19 (-198.6826, 24) -> (-24.7826, 24)
  line L20 (-6.7826, 0) -> (-183.8326, 0)
  line L21 (-183.8326, 0) -> (-6.7826, 0)
  line L22 (-6.7826, 0) -> (-6.7826, 12)
  line L23 (-1.224137, 12) -> (-24.7826, 12)
  line L24 (-94.974342, 0) -> (-74.890858, 0)
  line L25 (-94.974342, 24) -> (-94.974342, 0)
  line L26 (-94.974342, 0) -> (-6.7826, 0)
  line L27 (0, -2) -> (-198.6826, -2)
  point P0 (-198.6826, 48)
  point P1 (-94.974342, 12)
  point P2 (-6.7826, 11.809383)
  constraints: 32 end point, 4 collinear, 4 perpendicular, 4 point on line, 3 midpoint, 3 vertical, 1 horizontal, 1 parallel
extrude "Extrusion23" cut sketch "Sketch25" against normal through all contours L14 L13 L12 L11 L4 L3 L0 | L3 L4 L11 L22 L23 L8 L9 L6 L5 | L9 L18 L15 L16 | L11 L23 L22 | L9 L25 L15 L18 | L15 L25 L9 L8
sketch "Sketch26" plane through (230.9326, 42, -2) normal (0, 1, 0) x (1, 0, 0)
  line L0 (0, 0) -> (0, 11.737557)
  line L1 (0, 11.737557) -> (0, -2)
  line L2 (0, -2) -> (-198.6826, -2)
  line L3 (0, -2) -> (-198.6826, -2)
  line L4 (-198.6826, 12) -> (-198.6826, 0)
  line L5 (-198.6826, -2) -> (-198.6826, 12)
  line L6 (-198.6826, 12) -> (0, 11.737557)
  line L7 (-198.6826, 12) -> (-128.6826, 12)
  line L8 (-24.7826, 12) -> (-198.6826, 12)
  line L9 (-128.6826, 12) -> (-128.6826, -2)
  line L10 (-136.974342, -2) -> (-116.890858, -2)
  line L11 (-128.6826, -2) -> (-130.6826, -2)
  line L12 (-130.6826, -2) -> (-130.6826, 12)
  line L13 (-130.6826, 12) -> (0, 11.737557)
  line L14 (0, 11.737557) -> (-130.6826, 12)
  line L15 (-130.6826, 11.910178) -> (-130.6826, 15.270832)
  line L16 (-130.6826, 15.270832) -> (0, 15.270832)
  line L17 (0, 15.270832) -> (0, 11.737557)
  line L18 (0, -2) -> (-3, -2)
  line L19 (-3, -2) -> (-3, 15.270832)
  point P0 (-230.9326, -2)
  point P1 (-128.6826, 11.907536)
  point P2 (-128.6826, -2)
  point P3 (-128.6826, 11.995984)
  point P4 (-3, -2)
  point P5 (-3, 11.74152)
  dimension "d262" = 70
  dimension "d265" = 2
  dimension "d266" = 3
  constraints: 30 end point, 9 point on line, 5 perpendicular, 2 collinear, 1 parallel, 1 vertical
  measures "d262" distance of L4.start L7.end
  measures "d265" distance of L9.end L11.end
  measures "d266" distance of L1.end L18.end
extrude "Extrusion24" cut sketch "Sketch26" against normal blind 35 contours L6 L19 L16 L17 | L19 L2 L9 L6 | L6 L9 L13 | L13 L9 L7 L15 L16 L19
sketch "Sketch27" plane through (230.9326, 42, -2) normal (0, 1, 0) x (1, 0, 0)
  line L0 (-31.974342, -2) -> (0.275863, -2)
  line L1 (0.017866, -2) -> (-3.236092, -2)
  line L2 (-3.236092, -2) -> (-3.236092, 14.473652)
  line L3 (-3.236092, 14.473652) -> (0.017866, 14.473652)
  line L4 (0.017866, 14.473652) -> (0.017866, -2)
  line L5 (0.017866, -2) -> (20.642801, -2)
  line L6 (20.642801, -2) -> (20.642801, 14.745886)
  line L7 (20.642801, 14.745886) -> (0.017866, 14.745886)
  line L8 (0.017866, 14.745886) -> (0.017866, -2)
  point P0 (-230.9326, -2)
  constraints: 16 end point, 4 parallel, 2 horizontal, 2 perpendicular, 1 point on line
extrude "Extrusion25" cut sketch "Sketch27" against normal blind 27
sketch "Sketch28" plane through (230.9326, 42, -2) normal (0, 1, 0) x (1, 0, 0)
  line L0 (-183.8326, 0) -> (-179.890858, 0)
  line L1 (-183.8326, 0) -> (-185.8326, 0)
  line L2 (-185.8326, 0) -> (-185.8326, -2)
  line L3 (-219.357044, -2) -> (-179.890858, -2)
  line L4 (-230.9326, -2) -> (-228.9326, -2)
  line L5 (-185.8326, -2) -> (-230.9326, -2)
  line L6 (-230.9326, -2) -> (-185.8326, -2)
  line L7 (-185.8326, -2) -> (-185.8326, 12)
  line L8 (-198.6826, 12) -> (-179.890858, 12)
  line L9 (-185.8326, 12) -> (-230.9326, 12)
  line L10 (-230.9326, 48) -> (-230.9326, -2)
  line L11 (-230.9326, 12) -> (-230.9326, -2)
  line L12 (-185.8326, 12) -> (-230.9326, 12)
  line L13 (-230.9326, 12) -> (-230.9326, 48)
  line L14 (-230.9326, 48) -> (-185.8326, 48)
  line L15 (-185.8326, 48) -> (-185.8326, 12)
  dimension "d269" = 2
  constraints: 22 end point, 4 perpendicular, 4 point on line, 3 equal length, 3 horizontal
  measures "d269" distance of L0.start L1.end
extrude "Extrusion26" cut sketch "Sketch28" against normal blind 20
body "Solid1"
